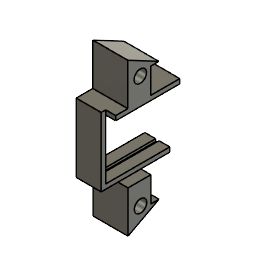
TwoSiPM_Metalens_Holder_LeftWindow_3Walls (Autodesk Fusion 360 design; units mm, degrees)
part number: 2026-07-09-10-14-52-773
Autodesk Fusion 360 part; units mm, degrees
sketch "Sketch Metalens Holder" plane through (0, 0, 0) normal (1, 0, 0) x (0, 0, -1)
  line L0 (0, 8.15) -> (16.5, 8.15)
  line L1 (16.5, 8.15) -> (16.5, -8.35)
  line L2 (16.5, -8.35) -> (0, -8.35)
  line L3 (0, -8.35) -> (0, 8.15)
  dimension "d3" = 16.5
  dimension "d4" = 16.5
  constraint perpendicular L0 L1
  constraint perpendicular L0 L3
  constraint vertical L3
  constraint horizontal L2
  measures "d3" distance of L0.start L0.end
  measures "d4" distance of L0.end L1.end
extrude "Extrude Metalens Holder" add sketch "Sketch Metalens Holder" along normal blind 6
shell "Shell Metalens Holder" thickness 1.1 removed faces 2 at (6, 2.65, -5.5) at (0, 2.65, -5.5)
sketch "Sketch Screwing Parts" plane through (0, 0, 0) normal (1, 0, 0) x (0, 0, -1)
  line L0 (4, 8.15) -> (4, 18.2)
  line L1 (4, 18.2) -> (11.49, 14.228)
  line L2 (11.49, 14.228) -> (9.515, 14.228)
  line L3 (9.515, 14.228) -> (9.515, 8.15)
  line L4 (4, 8.15) -> (9.515, 8.15)
  circle A0 centre (7, 13.4) radius 1.5
  line L5 (0, 8.15) -> (16.5, 8.15)
  line L6 (4.0564, -8.35) -> (4.0564, -18.4)
  line L7 (0.0564, -8.35) -> (16.5564, -8.35)
  line L8 (0, -8.35) -> (16.5, -8.35)
  line L9 (9.5564, -8.35) -> (9.5564, -14.428)
  line L10 (9.5564, -14.428) -> (11.5314, -14.428)
  line L11 (4.0564, -18.4) -> (11.5314, -14.428)
  circle A1 centre (7.0564, -13.6) radius 1.5
  point P0 (0, 8.15)
  dimension "d48" = 10.05
  dimension "d50" = 8.478
  dimension "d51" = 1.975
  dimension "d55" = 3
  dimension "d57" = 4.8
  dimension "d65" = 16.5
  dimension "d66" = 4
  dimension "d68" = 5.5
  dimension "d72" = 4.8
  dimension "d73" = 9.5
  dimension "d74" = 7
  dimension "d75" = 6.078
  dimension "d76" = 27
  dimension "d77" = 36.6
  constraint vertical L0
  constraint horizontal L2
  constraint perpendicular L2 L3
  constraint horizontal L4
  constraint horizontal L5
  constraint coincident L0.start L5
  constraint vertical L6
  constraint horizontal L7
  constraint coincident L6.start L7
  constraint coincident L6.start L8
  constraint coincident L8 L9.start
  constraint perpendicular L8 L9
  constraint perpendicular L9 L10
  constraint equal L0 L6
  constraint equal L3 L9
  constraint equal L2 L10
  measures "d48" distance of L0.start L0.end
  measures "d50" distance of L0.end L1.end
  measures "d51" distance of L1.end L2.end
  measures "d55" diameter of A0
  measures "d57" vertical distance of L0.end A0.centre
  measures "d65" distance of L7.start L7.end
  measures "d66" distance of L6.start L7.start
  measures "d68" distance of L6.start L9.start
  measures "d72" vertical distance of L6.end A1.centre
  measures "d73" horizontal distance of L7.end A1.centre
  measures "d74" horizontal distance of L7.start A1.centre
  measures "d75" distance of L9.start L9.end
  measures "d76" vertical distance of A0.centre A1.centre
  measures "d77" vertical distance of L0.end L6.end
extrude "Extrude Crewing Parts" add sketch "Sketch Screwing Parts" along normal blind 8.4
ref_plane "WorkPlane1" through (3, -0.1, -8.25) normal (-1, 0, 0) x (0, 0, 1)
sketch "Sketch Inside Slit" plane through (3, 0, 0) normal (-1, 0, 0) x (0, 0, 1)
  line L0 (-15.4, 7.05) -> (-15.4, -7.25)
  line L1 (-16, 7.65) -> (-0.5, 7.65)
  line L2 (-0.5, 7.65) -> (-0.5, -7.85)
  line L3 (-0.5, -7.85) -> (-16, -7.85)
  line L4 (-16, -7.85) -> (-16, 7.65)
  line L5 (-15.4, 7.05) -> (-1.1, 7.05)
  line L6 (-1.1, 7.05) -> (-1.1, -7.25)
  line L7 (-1.1, -7.25) -> (-15.4, -7.25)
  line L8 (-15.4, -7.25) -> (-15.4, 7.05)
  line L9 (-15.4, 7.05) -> (-16, 7.05)
  line L10 (-1.1, 7.05) -> (-0.5, 7.05)
  line L11 (-1.1, -7.25) -> (-0.5, -7.25)
  line L12 (-15.4, -7.25) -> (-16, -7.25)
  point P0 (-1.1, -7.25)
  point P1 (-1.1, 7.05)
  dimension "d91" = 15.5
  constraint horizontal L1
  constraint vertical L2
  constraint horizontal L3
  constraint vertical L4
  constraint equal L1 L4
  constraint coincident P0 L6.end
  constraint coincident P1 L5.end
  constraint horizontal L5
  constraint vertical L6
  constraint horizontal L7
  constraint vertical L8
  constraint coincident L0.start L5.start
  constraint coincident L4 L9.end
  constraint perpendicular L4 L9
  constraint coincident L2 L10.end
  constraint perpendicular L2 L10
  constraint coincident L2 L11.end
  constraint perpendicular L2 L11
  constraint coincident L0.end L7.end
  constraint coincident L4 L12.end
  constraint perpendicular L4 L12
  measures "d91" distance of L1.start L1.end
extrude "Extrude Inside Slit" cut sketch "Sketch Inside Slit" along normal mid plane 0.8 contours L2 L6 L10 L11
extrude "Extrude Inside Slit Bis" cut sketch "Sketch Inside Slit" along normal mid plane 0.8 contours L1 L2 L4 L5 L9 L10
extrude "Extrude Inside Slit BisBis" cut sketch "Sketch Inside Slit" along normal mid plane 0.8 contours L0 L4 L8 L9 L12
extrude "Extrude Inside Slit BisBisBis" cut sketch "Sketch Inside Slit" along normal mid plane 0.8
sketch "Sketch9" plane through (6, 0, 0) normal (1, 0, 0) x (0, 0, -1)
  line L0 (1.1, -7.25) -> (1.1, 7.05)
  line L1 (1.1, 7.05) -> (15.4, 7.05)
  line L2 (15.4, 7.05) -> (15.4, -7.25)
  line L3 (16.5, -8.35) -> (16.5, 8.15)
  line L4 (16.5, 8.15) -> (9.515, 8.15)
  line L5 (9.515, 8.15) -> (4, 8.15)
  line L6 (4, 8.15) -> (0, 8.15)
  line L7 (0, 8.15) -> (0, -8.35)
  line L8 (1.1, 8.15) -> (16.5, 8.15)
  line L9 (1.1, 7.05) -> (1.1, 8.15)
  line L10 (16.5, 8.15) -> (16.5, 7.05)
  line L11 (1.1, 7.05) -> (16.5, 7.05)
  line L12 (15.4, -7.25) -> (1.1, -7.25)
  line L13 (0, -8.35) -> (4.0564, -8.35)
  line L14 (4.0564, -8.35) -> (9.5564, -8.35)
  line L15 (9.5564, -8.35) -> (16.5, -8.35)
  dimension "d102" = 1.1
  dimension "d106" = 1.1
  constraint coincident L6 L8.start
  constraint coincident L3.end L4.start
  constraint coincident L1 L0.end
  constraint vertical L9
  constraint perpendicular L8 L10
  measures "d102" distance of L6.end L8.start
  measures "d106" distance of L3.end L10.end
extrude "ExtrudeÉchasse" add sketch "Sketch9" along normal blind 2.4 contours L1 L3 L4 L5 L6 L8 L9 L10 L11
extrude "Extrude" cut 1 faces at (0.8667, 2.2833, -15.4) along direction (0, 0, -1) blind 1.1
extrude "Extrude22" cut 1 faces at (4.2667, 2.2833, -15.4) along direction (0, 0, -1) blind 1.1
extrude "Extrude23" cut 1 faces at (3.1333, -2.4833, -16) along direction (0, 0, -1) blind 0.5
